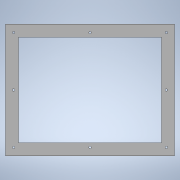
# Autodesk Inventor part: auth panel face plate seal
Saved by Autodesk Inventor 2022 (Build 260153000, 153)
## iProperties
Created: 2022-05-25
Part Number: auth panel face plate seal
Material: Generic
Document SubType Name: Modeling
Designer: alecw
Density: 1 g/cm^3
Appearance: Default
Author: alecw
Autodesk Inventor part; units mm, degrees
ref_plane "YZ Plane" through (0, 0, 0) normal (1, 0, 0) x (0, 1, 0)
ref_plane "XZ Plane" through (0, 0, 0) normal (0, 1, 0) x (-1, 0, 0)
ref_plane "Backplate Depth" through (0, 0, -3.2) normal (0, 0, 1) x (1, 0, 0)
sketch "Sketch2" plane through (0, 0, 0) normal (0, 0, 1) x (1, 0, 0)
  line L0 (0, 0) -> (49.8, 0)
  line L1 (49.8, 0) -> (49.8, 65)
  line L2 (49.8, 65) -> (0, 65)
  line L3 (0, 65) -> (0, 0)
  line L4 (0, 0) -> (-8.8, 0)
  line L5 (-8.8, 0) -> (-12, 0)
  line L6 (-12, 0) -> (-42, 0)
  line L7 (-42, 0) -> (-54.8, 0)
  line L8 (-54.8, 0) -> (-99.5, 0)
  line L9 (-99.5, 0) -> (-105.9, 0)
  line L10 (-105.9, 0) -> (-114.7, 0)
  line L11 (-114.7, 0) -> (-114.7, 40.1)
  line L12 (-114.7, 40.1) -> (0, 40.1)
  line L13 (-114.7, 0) -> (0, 0)
  line L14 (-105.9, 0) -> (-105.9, 40.1)
  line L15 (-8.8, 40.1) -> (-8.8, 0)
  line L16 (-48.4, 0) -> (-8.8, 0)
  line L17 (0, 65) -> (-114.7, 65)
  line L18 (-114.7, 65) -> (-114.7, 40.1)
  line L19 (49.8, 0) -> (54.6, 0)
  line L20 (0, 65) -> (0, 69.8)
  line L21 (0, 69.8) -> (54.6, 69.8)
  line L22 (54.6, 69.8) -> (54.6, 0)
  line L23 (-54.8, 0) -> (-48.4, 0)
  line L24 (-42, 0) -> (-48.4, 0)
  line L25 (-48.4, 0) -> (-48.4, 40.1)
  line L26 (-105.9, 40.1) -> (-105.9, 33.7)
  line L27 (-105.9, 40.1) -> (-93.1, 40.1)
  line L28 (-105.9, 0) -> (-48.4, 0)
  line L29 (-99.5, 0) -> (-88.19, 0)
  line L30 (-88.19, 0) -> (-79.22, 0)
  line L31 (-54.8, 0) -> (-54.8, 40.1)
  line L32 (-99.5, 0) -> (-99.5, 40.1)
  line L33 (-54.8, 40.1) -> (-56.9213, 37.9787)
  line L34 (-54.8, 40.1) -> (-51.8, 40.1) construction
  line L35 (-56.9213, 37.9787) -> (-54.8, 35.8574)
  line L36 (-56.9213, 37.9787) -> (-59.0426, 40.1)
  line L37 (-54.8, 0) -> (-57.6284, 2.8284)
  line L38 (-54.8, 0) -> (-50.8, 0) construction
  line L39 (-99.5, 40.1) -> (-95.9645, 36.5645)
  line L40 (-99.5, 40.1) -> (-94.5, 40.1) construction
  line L41 (-95.9645, 36.5645) -> (-92.4289, 40.1)
  line L42 (-95.9645, 36.5645) -> (-99.5, 33.0289)
  line L43 (-99.5, 0) -> (-95.9645, 3.5355)
  line L44 (-99.5, 0) -> (-94.5, 0) construction
  line L45 (-95.9645, 3.5355) -> (-92.4289, 0)
  line L46 (-95.9645, 3.5355) -> (-99.5, 7.0711)
  line L47 (-48.4, 0) -> (-48.4, -6.4)
  line L48 (-48.4, -6.4) -> (-105.9, -6.4)
  line L49 (-105.9, -6.4) -> (-105.9, 0)
  line L50 (-105.9, 40.1) -> (-105.9, 46.5)
  line L51 (-48.4, 40.1) -> (-48.4, 46.5)
  line L52 (-48.4, 46.5) -> (-105.9, 46.5)
  line L53 (-88.19, 0) -> (-86.59, 0)
  line L54 (-88.19, 0) -> (-89.79, 0)
  line L55 (-89.79, 0) -> (-86.59, 0)
  line L56 (-86.59, 0) -> (-86.59, 40.1)
  line L57 (-86.59, 40.1) -> (-89.79, 40.1)
  line L58 (-89.79, 40.1) -> (-89.79, 0)
  line L59 (-80.82, 40.1) -> (-80.82, 0)
  line L60 (-77.62, 0) -> (-77.62, 40.1)
  line L61 (-71.85, 40.1) -> (-71.85, 0)
  line L62 (-68.65, 0) -> (-68.65, 40.1)
  line L63 (-62.88, 40.1) -> (-62.88, 0)
  line L64 (-59.68, 0) -> (-59.68, 40.1)
  line L65 (0, 0) -> (0, -6.4)
  line L66 (0, -6.4) -> (0, -15.2)
  line L67 (-114.7, 0) -> (-114.7, -6.4)
  line L68 (-114.7, -6.4) -> (-114.7, -15.2)
  line L69 (-114.7, -15.2) -> (0, -15.2)
  line L70 (0, -15.2) -> (54.6, -15.2)
  line L71 (54.6, -15.2) -> (54.6, 0)
  line L72 (-28.6, 40.1) -> (-28.6, 0)
  circle A0 centre (-28.6, 20.05) radius 9.5
  circle A1 centre (-28.6, 20.05) radius 10.5
  line L73 (-28.6, 29.55) -> (-27.303, 29.4611)
  line L74 (-27.303, 29.4611) -> (-27.2345, 30.4608)
  line L75 (-28.6, 29.55) -> (-29.897, 29.4611)
  line L76 (-29.897, 29.4611) -> (-29.9655, 30.4608)
  line L77 (-105.9, 46.5) -> (-114.7, 46.5)
  line L78 (-105.9, -6.4) -> (-114.7, -6.4)
  line L79 (-48.4, -6.4) -> (0, -6.4)
  line L80 (-28.6, 20.05) -> (-35, 20.05)
  line L81 (-28.6, 20.05) -> (-22.2, 20.05)
  circle A2 centre (-28.6, 20.05) radius 14.7
  line L82 (-77.62, 40.1) -> (-71.85, 40.1)
  line L83 (-88.19, 40.1) -> (-92.19, 40.1)
  line L84 (-92.19, 40.1) -> (-93.79, 40.1)
  line L85 (-74.735, 0) -> (-74.735, 40.1)
  line L86 (-92.135, 38.25) -> (-57.335, 38.25)
  line L87 (-57.335, 38.25) -> (-57.335, 1.85)
  line L88 (-57.335, 1.85) -> (-92.135, 1.85)
  line L89 (-92.135, 1.85) -> (-92.135, 38.25)
  line L90 (-92.135, 38.25) -> (-57.335, 1.85) construction
  line L91 (-57.335, 38.25) -> (-92.135, 1.85) construction
  line L92 (-74.735, 38.25) -> (-74.735, 40.1)
  line L93 (-18.1, 20.05) -> (-17.1, 20.05)
  circle A3 centre (-28.6, 20.05) radius 11.5
  line L94 (-17.1, 20.05) -> (-13.9, 20.05)
  line L95 (-54.8, 40.1) -> (-48.4, 40.1)
  line L96 (-89.79, 38.25) -> (-86.59, 38.25)
  line L97 (-59.68, 38.25) -> (-62.88, 38.25)
  line L98 (-92.135, 20.05) -> (-57.335, 20.05)
  line L99 (-57.6284, 2.8284) -> (-54.8, 5.6569)
  line L100 (-57.6284, 2.8284) -> (-60.4569, 0)
  line L101 (-99.5, 20.05) -> (-105.9, 20.05)
  circle A4 centre (-102.7, 20.05) radius 0.9
  line L102 (-54.8, 20.05) -> (-48.4, 20.05)
  circle A5 centre (-51.6, 20.05) radius 0.9
  line L103 (0, -15.2) -> (0, -20)
  line L104 (0, -20) -> (-114.7, -20)
  line L105 (-114.7, -20) -> (-114.7, -15.2)
  line L106 (-88.19, 40.1) -> (-88.19, 43.3)
  circle A6 centre (-88.19, 43.3) radius 0.9
  circle A7 centre (-61.28, 43.3) radius 0.9
  line L107 (-102.7, 20.05) -> (-102.7, 0)
  circle A8 centre (-102.7, 10.025) radius 0.9
  circle A9 centre (-102.7, 30.075) radius 0.9
  circle A10 centre (-51.6, 30.075) radius 0.9
  circle A11 centre (-51.6, 10.025) radius 0.9
  line L108 (0, -20) -> (54.6, -20)
  line L109 (54.6, -20) -> (54.6, -15.2)
  line L110 (0, 65) -> (0, 73.8)
  line L111 (0, 73.8) -> (-114.7, 73.8)
  line L112 (-114.7, 73.8) -> (-114.7, 65)
  line L113 (-105.9, -20) -> (-105.9, 73.8)
  line L114 (-8.8, -20) -> (-8.8, 73.8)
  line L115 (-28.6, 40.1) -> (-48.4, 40.1)
  line L116 (-28.6, 40.1) -> (-8.8, 40.1)
  line L117 (-48.4, 46.5) -> (-28.6, 46.5)
  line L118 (-28.6, 46.5) -> (-8.8, 46.5)
  line L119 (-28.6, 46.5) -> (-28.6, 65)
  line L120 (-25.4, 52.55) -> (-31.8, 52.55)
  line L121 (-31.8, 52.55) -> (-31.8, 58.95)
  line L122 (-31.8, 58.95) -> (-25.4, 58.95)
  line L123 (-25.4, 58.95) -> (-25.4, 52.55)
  line L124 (-25.4, 52.55) -> (-31.8, 58.95) construction
  line L125 (-31.8, 52.55) -> (-25.4, 58.95) construction
  line L126 (-24.1, 51.25) -> (-33.1, 51.25)
  line L127 (-33.1, 51.25) -> (-33.1, 60.25)
  line L128 (-33.1, 60.25) -> (-24.1, 60.25)
  line L129 (-24.1, 60.25) -> (-24.1, 51.25)
  line L130 (-24.1, 51.25) -> (-33.1, 60.25) construction
  line L131 (-33.1, 51.25) -> (-24.1, 60.25) construction
  line L132 (-25.4, 52.55) -> (-25.4, 51.25)
  line L133 (-31.8, 52.55) -> (-31.8, 51.25)
  circle A12 centre (-88.19, 43.3) radius 2.4
  circle A13 centre (-61.28, 43.3) radius 2.4
  circle A14 centre (-51.6, 30.075) radius 2.4
  circle A15 centre (-51.6, 20.05) radius 2.4
  circle A16 centre (-102.7, 10.025) radius 2.4
  circle A17 centre (-102.7, 20.05) radius 2.4
  circle A18 centre (-102.7, 30.075) radius 2.4
  line L134 (-114.7, -20) -> (-114.7, -22.4)
  line L135 (-114.7, -22.4) -> (-117.1, -22.4)
  line L136 (-114.7, -15.2) -> (-114.7, -12.8)
  line L137 (-114.7, -12.8) -> (-112.3, -12.8)
  line L138 (0, 73.8) -> (-2.4, 73.8)
  line L139 (-2.4, 73.8) -> (-2.4, 71.4)
  line L140 (-112.3, -12.8) -> (-112.3, 71.4)
  line L141 (-112.3, 71.4) -> (-2.4, 71.4)
  line L142 (-2.4, 71.4) -> (-2.4, -12.8)
  line L143 (-2.4, -12.8) -> (-112.3, -12.8)
  line L144 (-2.4, -15.2) -> (-2.4, -12.8)
  line L145 (-28.6, -6.4) -> (-28.6, 0)
  circle A19 centre (-28.6, -3.2) radius 2.4
  circle A20 centre (-28.6, -3.2) radius 0.9
  line L146 (-28.6, 40.1) -> (-28.6, 46.5)
  circle A21 centre (-28.6, 43.3) radius 0.9
  circle A22 centre (-28.6, 43.3) radius 2.4
  line L147 (-105.9, 65) -> (-105.9, 71.4)
  circle A23 centre (-109.1, 68.2) radius 0.9
  circle A24 centre (-109.1, 68.2) radius 2
  line L148 (-8.8, 65) -> (-2.4, 65)
  line L149 (-8.8, -6.4) -> (-8.8, -12.8)
  line L150 (-105.9, 65) -> (-112.3, 65)
  line L151 (-105.9, 65) -> (-105.9, 71.4)
  line L152 (-105.9, 68.2) -> (-109.1, 68.2)
  line L153 (-109.1, 65) -> (-109.1, 68.2)
  line L154 (-105.9, -6.4) -> (-105.9, -12.8)
  circle A25 centre (-57.35, 68.2) radius 2
  circle A26 centre (-57.35, 68.2) radius 0.9
  circle A27 centre (-5.6, 68.2) radius 2
  circle A28 centre (-5.6, 68.2) radius 0.9
  circle A29 centre (-109.1, -9.6) radius 2
  circle A30 centre (-109.1, -9.6) radius 0.9
  circle A31 centre (-57.35, -9.6) radius 2
  circle A32 centre (-57.35, -9.6) radius 0.9
  circle A33 centre (-5.6, -9.6) radius 2
  circle A34 centre (-5.6, -9.6) radius 0.9
  line L155 (-105.9, -6.4) -> (-105.9, 65)
  line L156 (-105.9, 29.3) -> (-112.3, 29.3)
  circle A35 centre (-109.1, 29.3) radius 2
  circle A36 centre (-109.1, 29.3) radius 0.9
  circle A37 centre (-5.6, 29.3) radius 0.9
  circle A38 centre (-5.6, 29.3) radius 2
  line L157 (-105.9, 29.3) -> (-105.9, 65)
  line L158 (-8.8, 65) -> (-105.9, 65)
  line L159 (-57.35, 65) -> (-109.1, 65)
  circle A39 centre (-109.1, 68.2) radius 1.6
  circle A40 centre (-97.6, 68.2) radius 1.6
  circle A41 centre (-86.1, 68.2) radius 1.6
  circle A42 centre (-74.6, 68.2) radius 1.6
  circle A43 centre (-63.1, 68.2) radius 1.6
  circle A44 centre (-51.6, 68.2) radius 1.6
  circle A45 centre (-40.1, 68.2) radius 1.6
  circle A46 centre (-28.6, 68.2) radius 1.6
  circle A47 centre (-17.1, 68.2) radius 1.6
  circle A48 centre (-109.1, 57.0857) radius 1.6
  circle A49 centre (-109.1, 45.9714) radius 1.6
  circle A50 centre (-109.1, 34.8571) radius 1.6
  circle A51 centre (-109.1, 23.7429) radius 1.6
  circle A52 centre (-109.1, 12.6286) radius 1.6
  circle A53 centre (-109.1, 1.5143) radius 1.6
  line L160 (-57.35, 65) -> (-57.35, 71.4)
  circle A54 centre (-97.6, -9.6) radius 1.6
  circle A55 centre (-86.1, -9.6) radius 1.6
  circle A56 centre (-74.6, -9.6) radius 1.6
  circle A57 centre (-63.1, -9.6) radius 1.6
  circle A58 centre (-51.6, -9.6) radius 1.6
  circle A59 centre (-40.1, -9.6) radius 1.6
  circle A60 centre (-28.6, -9.6) radius 1.6
  circle A61 centre (-17.1, -9.6) radius 1.6
  circle A62 centre (-5.6, 57.0857) radius 1.6
  circle A63 centre (-5.6, 45.9714) radius 1.6
  circle A64 centre (-5.6, 34.8571) radius 1.6
  circle A65 centre (-5.6, 23.7429) radius 1.6
  circle A66 centre (-5.6, 12.6286) radius 1.6
  circle A67 centre (-5.6, 1.5143) radius 1.6
  line L161 (-48.4, 46.5) -> (-48.4, 65)
  line L162 (-92.135, 38.25) -> (-92.985, 38.25)
  line L163 (-92.985, 38.25) -> (-92.985, 39.1)
  line L164 (-56.485, 1) -> (-92.985, 1)
  line L165 (-92.985, 1) -> (-92.985, 39.1)
  line L166 (-92.985, 39.1) -> (-56.485, 39.1)
  line L167 (-56.485, 39.1) -> (-56.485, 1)
  line L168 (-56.485, 1) -> (-92.985, 39.1) construction
  line L169 (-92.985, 1) -> (-56.485, 39.1) construction
  line L170 (-92.985, 39.1) -> (-92.985, 40.1)
  line L171 (-92.985, 40.1) -> (-93.985, 40.1)
  line L172 (-55.485, 0) -> (-93.985, 0)
  line L173 (-93.985, 0) -> (-93.985, 40.1)
  line L174 (-93.985, 40.1) -> (-55.485, 40.1)
  line L175 (-55.485, 40.1) -> (-55.485, 0)
  line L176 (-55.485, 0) -> (-93.985, 40.1) construction
  line L177 (-93.985, 0) -> (-55.485, 40.1) construction
  line L178 (54.6, -20) -> (59.6, -20)
  line L179 (59.6, -20) -> (59.6, 69.8)
  line L180 (59.6, 69.8) -> (54.6, 69.8)
  line L181 (59.6, -20) -> (61.6, -20)
  line L182 (61.6, -20) -> (61.6, 69.8)
  line L183 (61.6, 69.8) -> (59.6, 69.8)
  line L184 (59.6, 65) -> (61.6, 65)
  line L185 (59.6, -20) -> (59.6, -16.8)
  line L186 (59.6, -16.8) -> (61.6, -16.8)
  line L187 (-8.8, -20) -> (-105.9, -20)
  line L188 (-105.9, -20) -> (-101.9, -20)
  line L189 (-57.35, -20) -> (-57.35, -15.2)
  line L190 (-101.9, -20) -> (-101.4, -20)
  line L191 (-101.4, -20) -> (-93.4, -20)
  line L192 (-93.4, -20) -> (-93.4, -15.2)
  line L193 (-101.9, -20) -> (-101.9, -15.2)
  line L194 (-101.4, -20) -> (-101.4, -15.2)
  line L195 (-93.4, -20) -> (-92.9, -20)
  line L196 (-92.9, -20) -> (-84.9, -20)
  line L197 (-84.9, -20) -> (-84.9, -15.2)
  line L198 (-8.8, -20) -> (-12.8, -20)
  line L199 (-12.8, -20) -> (-13.3, -20)
  line L200 (-13.3, -20) -> (-21.3, -20)
  line L201 (-21.3, -20) -> (-21.3, -15.2)
  line L202 (-12.8, -20) -> (-12.8, -15.2)
  line L203 (-13.3, -20) -> (-13.3, -15.2)
  line L204 (-21.3, -20) -> (-21.8, -20)
  line L205 (-21.8, -20) -> (-29.8, -20)
  line L206 (-29.8, -20) -> (-29.8, -15.2)
  line L207 (-57.35, 73.8) -> (-57.35, 75.8)
  line L208 (-57.35, 75.8) -> (-77.35, 75.8)
  line L209 (-77.35, 75.8) -> (-79.35, 73.8)
  line L210 (-77.35, 75.8) -> (-74.5216, 75.8) construction
  line L211 (-57.35, 75.8) -> (-37.35, 75.8)
  line L212 (-37.35, 75.8) -> (-35.35, 73.8)
  line L213 (0, 73.8) -> (61.6, 73.8)
  line L214 (61.6, 73.8) -> (61.6, 69.8)
  line L215 (0, 73.8) -> (0.5, 73.8)
  line L216 (0.5, 73.8) -> (0.5, -20)
  line L217 (59.6, 69.8) -> (59.6, 73.8)
  line L218 (54.6, -15.2) -> (61.6, -15.2)
  line L219 (-92.9, -20) -> (-92.9, -15.2)
  line L220 (-21.8, -20) -> (-21.8, -15.2)
  line L221 (0.5, -15.2) -> (0.5, -10.4)
  line L222 (0.5, -10.4) -> (54.6, -10.4)
  line L223 (0.5, -15.2) -> (0.5, -10.4)
  line L224 (0.5, -10.4) -> (54.6, -10.4)
  line L225 (49.8, 0) -> (49.8, -15.2)
  line L226 (49.8, 69.8) -> (49.8, 65)
  line L227 (54.6, 65) -> (49.8, 65)
  line L228 (0.5, -15.2) -> (5.3, -15.2)
  line L229 (5.3, -15.2) -> (5.3, 65)
  line L230 (54.6, 69.8) -> (54.6, 73.8)
  line L231 (49.8, 69.8) -> (49.8, 73.8)
  line L232 (49.8, -15.2) -> (49.8, -20)
  line L233 (5.3, -15.2) -> (5.3, -20)
  line L234 (5.3, 65) -> (5.3, 73.8)
  line L235 (54.6, -10.4) -> (61.6, -10.4)
  line L236 (61.6, 65) -> (54.6, 65)
  line L237 (-35, 20.05) -> (-35, 13.0293)
  line L238 (-35, 20.05) -> (-35, 27.0707)
  line L239 (-22.2, 20.05) -> (-22.2, 27.0707)
  line L240 (-22.2, 20.05) -> (-22.2, 13.0293)
  line L241 (0, -6.4) -> (61.6, -6.4)
  line L242 (0, 0) -> (61.6, 0)
  line L243 (-35, 27.0707) -> (-35, 33.2837)
  line L244 (-22.2, 27.0707) -> (-22.2, 33.2837)
  line L245 (-27.303, 10.6389) -> (-27.2345, 9.6392)
  line L246 (-29.897, 10.6389) -> (-29.9655, 9.6392)
  line L247 (-35, 20.05) -> (-35, 6.8163)
  line L248 (-22.2, 20.05) -> (-22.2, 6.8163)
  line L249 (-99.5, 33.0289) -> (-101.5, 33.0289)
  line L250 (-92.4289, 40.1) -> (-92.4289, 42.1)
  line L251 (-92.4289, 42.1) -> (-101.5, 42.1)
  line L252 (-101.5, 42.1) -> (-101.5, 33.0289)
  line L253 (-99.5, 7.0711) -> (-101.5, 7.0711)
  line L254 (-92.4289, 0) -> (-92.4289, -2)
  line L255 (-92.4289, -2) -> (-101.5, -2)
  line L256 (-101.5, -2) -> (-101.5, 7.0711)
  line L257 (-54.8, 5.6569) -> (-52.8, 5.6569)
  line L258 (-60.4569, 0) -> (-60.4569, -2)
  line L259 (-60.4569, -2) -> (-52.8, -2)
  line L260 (-52.8, -2) -> (-52.8, 5.6569)
  line L261 (-59.0426, 40.1) -> (-59.0426, 42.1)
  line L262 (-54.8, 35.8574) -> (-52.8, 35.8574)
  line L263 (-52.8, 35.8574) -> (-52.8, 42.1)
  line L264 (-52.8, 42.1) -> (-59.0426, 42.1)
  line L265 (-28.6, 52.55) -> (-30.1, 52.55)
  line L266 (-30.1, 52.55) -> (-30.1, 51.25)
  line L267 (-28.6, 52.55) -> (-27.1, 52.55)
  line L268 (-27.1, 52.55) -> (-27.1, 51.25)
  line L269 (-2.4, 29.3) -> (-2.4, 32.5)
  line L270 (-2.4, 32.5) -> (-8.8, 32.5)
  line L271 (-2.4, 29.3) -> (-2.4, 26.1)
  line L272 (-2.4, 26.1) -> (-8.8, 26.1)
  line L273 (-27.1, 58.95) -> (-27.1, 60.25)
  line L274 (-30.1, 58.95) -> (-30.1, 60.25)
  line L275 (-31.8, 58.95) -> (-31.8, 62.15)
  line L276 (-31.8, 62.15) -> (-35, 62.15)
  line L277 (-22.2, 49.35) -> (-35, 49.35)
  line L278 (-35, 49.35) -> (-35, 62.15)
  line L279 (-35, 62.15) -> (-22.2, 62.15)
  line L280 (-22.2, 62.15) -> (-22.2, 49.35)
  line L281 (-22.2, 49.35) -> (-35, 62.15) construction
  line L282 (-35, 49.35) -> (-22.2, 62.15) construction
  line L283 (-31.8, 58.95) -> (-32.1, 58.95)
  line L284 (-32.1, 58.95) -> (-32.1, 59.25)
  line L285 (-25.1, 52.25) -> (-32.1, 52.25)
  line L286 (-32.1, 52.25) -> (-32.1, 59.25)
  line L287 (-32.1, 59.25) -> (-25.1, 59.25)
  line L288 (-25.1, 59.25) -> (-25.1, 52.25)
  line L289 (-25.1, 52.25) -> (-32.1, 59.25) construction
  line L290 (-32.1, 52.25) -> (-25.1, 59.25) construction
  line L291 (-28.6, 55.75) -> (-28.6, 52.55)
  line L292 (-44.6, 52.55) -> (-38.2, 52.55)
  line L293 (-38.2, 52.55) -> (-38.2, 58.95)
  line L294 (-38.2, 58.95) -> (-44.6, 58.95)
  line L295 (-44.6, 58.95) -> (-44.6, 52.55)
  line L296 (-44.6, 52.55) -> (-38.2, 58.95) construction
  line L297 (-38.2, 52.55) -> (-44.6, 58.95) construction
  line L298 (-45.9, 51.25) -> (-36.9, 51.25)
  line L299 (-36.9, 51.25) -> (-36.9, 60.25)
  line L300 (-36.9, 60.25) -> (-45.9, 60.25)
  line L301 (-45.9, 60.25) -> (-45.9, 51.25)
  line L302 (-45.9, 51.25) -> (-36.9, 60.25) construction
  line L303 (-36.9, 51.25) -> (-45.9, 60.25) construction
  line L304 (-44.6, 52.55) -> (-44.6, 51.25)
  line L305 (-38.2, 52.55) -> (-38.2, 51.25)
  line L306 (-41.4, 52.55) -> (-39.9, 52.55)
  line L307 (-39.9, 52.55) -> (-39.9, 51.25)
  line L308 (-41.4, 52.55) -> (-42.9, 52.55)
  line L309 (-42.9, 52.55) -> (-42.9, 51.25)
  line L310 (-42.9, 58.95) -> (-42.9, 60.25)
  line L311 (-39.9, 58.95) -> (-39.9, 60.25)
  line L312 (-38.2, 58.95) -> (-38.2, 62.15)
  line L313 (-38.2, 62.15) -> (-35, 62.15)
  line L314 (-47.8, 49.35) -> (-35, 49.35)
  line L315 (-35, 62.15) -> (-47.8, 62.15)
  line L316 (-47.8, 62.15) -> (-47.8, 49.35)
  line L317 (-47.8, 49.35) -> (-35, 62.15) construction
  line L318 (-35, 49.35) -> (-47.8, 62.15) construction
  line L319 (-38.2, 58.95) -> (-37.9, 58.95)
  line L320 (-37.9, 58.95) -> (-37.9, 59.25)
  line L321 (-44.9, 52.25) -> (-37.9, 52.25)
  line L322 (-37.9, 52.25) -> (-37.9, 59.25)
  line L323 (-37.9, 59.25) -> (-44.9, 59.25)
  line L324 (-44.9, 59.25) -> (-44.9, 52.25)
  line L325 (-44.9, 52.25) -> (-37.9, 59.25) construction
  line L326 (-37.9, 52.25) -> (-44.9, 59.25) construction
  line L327 (-41.4, 55.75) -> (-41.4, 52.55)
  line L328 (-15.8, 46.5) -> (-15.8, 65)
  line L329 (-19, 52.55) -> (-12.6, 52.55)
  line L330 (-12.6, 52.55) -> (-12.6, 58.95)
  line L331 (-12.6, 58.95) -> (-19, 58.95)
  line L332 (-19, 58.95) -> (-19, 52.55)
  line L333 (-19, 52.55) -> (-12.6, 58.95) construction
  line L334 (-12.6, 52.55) -> (-19, 58.95) construction
  line L335 (-20.3, 51.25) -> (-11.3, 51.25)
  line L336 (-11.3, 51.25) -> (-11.3, 60.25)
  line L337 (-11.3, 60.25) -> (-20.3, 60.25)
  line L338 (-20.3, 60.25) -> (-20.3, 51.25)
  line L339 (-20.3, 51.25) -> (-11.3, 60.25) construction
  line L340 (-11.3, 51.25) -> (-20.3, 60.25) construction
  line L341 (-19, 52.55) -> (-19, 51.25)
  line L342 (-12.6, 52.55) -> (-12.6, 51.25)
  line L343 (-15.8, 52.55) -> (-14.3, 52.55)
  line L344 (-14.3, 52.55) -> (-14.3, 51.25)
  line L345 (-15.8, 52.55) -> (-17.3, 52.55)
  line L346 (-17.3, 52.55) -> (-17.3, 51.25)
  line L347 (-17.3, 58.95) -> (-17.3, 60.25)
  line L348 (-14.3, 58.95) -> (-14.3, 60.25)
  line L349 (-12.6, 58.95) -> (-12.6, 62.15)
  line L350 (-12.6, 62.15) -> (-9.4, 62.15)
  line L351 (-22.2, 49.35) -> (-9.4, 49.35)
  line L352 (-9.4, 49.35) -> (-9.4, 62.15)
  line L353 (-9.4, 62.15) -> (-22.2, 62.15)
  line L354 (-22.2, 49.35) -> (-9.4, 62.15) construction
  line L355 (-9.4, 49.35) -> (-22.2, 62.15) construction
  line L356 (-12.6, 58.95) -> (-12.3, 58.95)
  line L357 (-12.3, 58.95) -> (-12.3, 59.25)
  line L358 (-19.3, 52.25) -> (-12.3, 52.25)
  line L359 (-12.3, 52.25) -> (-12.3, 59.25)
  line L360 (-12.3, 59.25) -> (-19.3, 59.25)
  line L361 (-19.3, 59.25) -> (-19.3, 52.25)
  line L362 (-19.3, 52.25) -> (-12.3, 59.25) construction
  line L363 (-12.3, 52.25) -> (-19.3, 59.25) construction
  line L364 (-15.8, 55.75) -> (-15.8, 52.55)
  line L365 (-77.15, 46.5) -> (-77.15, 65)
  line L366 (5.3, -15.2) -> (5.3, -10.4)
  line L367 (0.5, -10.4) -> (5.3, -10.4)
  line L368 (5.3, -12.8) -> (2.9, -12.8)
  line L369 (2.9, -12.8) -> (2.9, -10.4)
  circle A68 centre (2.9, -12.8) radius 1
  circle A69 centre (2.9, -12.8) radius 0.9
  line L370 (54.6, -10.4) -> (49.8, -10.4)
  line L371 (52.2, -10.4) -> (2.9, -10.4)
  line L372 (5.3, 66.25) -> (5.3, -12.8)
  circle A70 centre (2.9, -12.8) radius 1.6
  line L373 (5.3, 69.8) -> (5.3, 65)
  line L374 (5.3, 67.4) -> (5.3, -12.8)
  line L375 (2.9, -10.4) -> (52.2, -10.4)
  point P0 (-74.735, 20.05)
  point P1 (-74.735, 20.05)
  point P2 (-112.3, 0)
  point P3 (-8.8, 71.4)
  point P4 (0.5, 0)
  point P5 (0, 69.8)
  point P6 (59.6, -15.2)
  point P7 (-8.8, -15.2)
  point P8 (-105.9, -15.2)
  point P9 (5.3, 0)
  point P10 (54.6, 0)
  point P11 (59.6, 0)
  point P12 (59.6, 65)
  point P13 (-60.4569, 0)
  point P14 (-60.4569, 0)
  point P15 (-92.4289, 0)
  point P16 (-68.65, 38.25)
  point P17 (-71.85, 38.25)
  point P18 (-71.85, 1.85)
  point P19 (-68.65, 1.85)
  point P20 (-62.88, 1.85)
  point P21 (-59.68, 1.85)
  point P22 (-80.82, 1.85)
  point P23 (-77.62, 1.85)
  point P24 (-77.62, 38.25)
  point P25 (-80.82, 38.25)
  point P26 (-86.59, 38.25)
  point P27 (-89.79, 1.85)
  point P28 (-86.59, 1.85)
  point P29 (-92.4289, 0)
  point P30 (-60.4569, 0)
  point P31 (49.8, -6.4)
  point P32 (5.3, -6.4)
  dimension "d1" = 49.8
  dimension "d2" = 65
  dimension "d3" = 8.8
  dimension "d4" = 3.2
  dimension "d5" = 30
  dimension "d6" = 12.8
  dimension "d7" = 44.7
  dimension "d11" = 40.1
  dimension "d15" = 4.8
  dimension "d16" = 4.8
  dimension "d21" = 11.31
  dimension "d22" = 8.97
  dimension "d23" = 3
  dimension "d24" = 135
  dimension "d25" = 4
  dimension "d26" = 135
  dimension "d27" = 5
  dimension "d28" = 45
  dimension "d29" = 5
  dimension "d30" = 45
  dimension "d33" = 6.4
  dimension "d34" = 1.6
  dimension "d35" = 1.6
  dimension "d38" = 8.97
  dimension "d43" = 3.2
  dimension "d45" = 19
  dimension "d46" = 21
  dimension "d47" = 1.3
  dimension "d48" = 6.4
  dimension "d49" = 6.4
  dimension "d53" = 4
  dimension "d54" = 1.6
  dimension "d55" = 34.8
  dimension "d56" = 36.4
  dimension "d59" = 1
  dimension "d61" = 3.2
  dimension "d70" = 1.8
  dimension "d71" = 1.8
  dimension "d72" = 4.8
  dimension "d74" = 3.2
  dimension "d75" = 1.8
  dimension "d76" = 1.8
  dimension "d79" = 51.1
  dimension "d86" = 6.4
  dimension "d88" = 9
  dimension "d89" = 4.8
  dimension "d98" = 2.4
  dimension "d99" = 2.4
  dimension "d100" = 2.4
  dimension "d101" = 2.4
  dimension "d102" = 2.4
  dimension "d103" = 2.4
  dimension "d104" = 2.4
  dimension "d105" = 1.8
  dimension "d106" = 4
  dimension "d109" = 51.75
  dimension "d116" = 77.8
  dimension "d123" = 38.9
  dimension "d128" = 3.2
  dimension "d131" = 11.5
  dimension "d138" = 11.1143
  dimension "d143" = 0.85
  dimension "d144" = 0.85
  dimension "d145" = 1
  constraints: 748 end point, 146 point on line, 94 symmetric about line, 71 centre point, 70 perpendicular, 65 midpoint, 55 horizontal, 45 vertical, 37 parallel, 26 coincident, 23 collinear, 15 point on circle, 14 horizontal alignment, 12 equal radius, 5 equal length, 96 other
  measures "d1" distance of L2.end L1.end
  measures "d2" distance of L1.end L0.end
  measures "d3" distance of L0.start L4.end
  measures "d4" distance of L4.end L5.end
  measures "d5" distance of L5.end L6.end
  measures "d6" distance of L6.end L7.end
  measures "d7" distance of L7.end L8.end
  measures "d11" distance of L10.end L11.end
  measures "d15" distance of L0.end L19.end
  measures "d16" distance of L2.end L20.end
  measures "d21" distance of L8.end L29.end
  measures "d22" distance of L29.end L30.end
  measures "d23" distance of L31.end L33.end
  measures "d24" angle of L33 L34
  measures "d25" distance of L7.end L37.end
  measures "d26" angle of L38 L37
  measures "d27" distance of L32.end L39.end
  measures "d28" angle of L39 L40
  measures "d29" distance of L8.end L43.end
  measures "d30" angle of L44 L43
  measures "d33" distance of L25.end L51.end
  measures "d34" distance of L29.end L53.end
  measures "d35" distance of L29.end L54.end
  measures "d38" distance of L57.end L59.start
  measures "d43" distance between parallel lines of L56 L58
  measures "d45" diameter of A0
  measures "d46" diameter of A1
  measures "d47" distance of L73.start L73.end
  measures "d48" distance of L80.start L80.end
  measures "d49" distance of L80.start L81.end
  measures "d53" distance of L83.start L83.end
  measures "d54" distance of L83.end L84.end
  measures "d55" distance of L87.end L88.end
  measures "d56" distance of L86.end L87.end
  measures "d59" distance of L93.start L93.end
  measures "d61" distance of L94.start L94.end
  measures "d70" diameter of A4
  measures "d71" diameter of A5
  measures "d72" distance of L66.end L103.end
  measures "d74" distance of L83.start L106.end
  measures "d75" diameter of A6
  measures "d76" diameter of A8
  measures "d79" distance of A9.centre A10.centre
  measures "d86" distance of L121.end L122.end
  measures "d88" distance of L126.end L127.end
  measures "d89" diameter of A12
  measures "d98" distance of L104.end L134.end
  measures "d99" distance of L134.end L135.end
  measures "d100" distance of L68.end L136.end
  measures "d101" distance of L136.end L137.end
  measures "d102" distance of L110.end L138.end
  measures "d103" distance of L138.end L139.end
  measures "d104" distance of L144.start L142.end
  measures "d105" diameter of A23
  measures "d106" diameter of A24
  measures "d109" distance of L152.end A25.centre
  measures "d116" distance of L152.end A29.centre
  measures "d123" distance of L152.end A35.centre
  measures "d128" diameter of A39
  measures "d131" distance of A39.centre A40.centre
  measures "d138" distance of A39.centre A48.centre
  measures "d143" distance of L86.start L162.end
  measures "d144" distance of L162.end L163.end
  measures "d145" distance of L163.end L170.end
ref_plane "Face Plate Start" through (0, 0, 5) normal (0, 0, 1) x (1, 0, 0)
ref_plane "TPU Seal Start" through (0, 0, 4) normal (0, 0, 1) x (1, 0, 0)
ref_plane "Face Plate End" through (0, 0, 8.2) normal (0, 0, 1) x (1, 0, 0)
ref_plane "Cover Clearance" through (0, 0, 11.2) normal (0, 0, 1) x (1, 0, 0)
ref_plane "Cover End" through (0, 0, 13.6) normal (0, 0, 1) x (1, 0, 0)
ref_plane "RFID Cover Start" through (0, 0, 12) normal (0, 0, 1) x (1, 0, 0)
extrude "Extrusion17" add sketch "Sketch2" along normal blind 0.6 contours L4 L142 L12 L3 | L65 L79 L142 L4 | L12 L142 L17 L3 | L142 L79 L114 L4 A67 | L4 A67 L15 L272 L142 | L66 L69 L144 L142 L79 | L17 L142 L139 L111 L110 L20 | L142 L270 L15 L12 | L12 L114 L17 L142 | A67 L4 | L4 A67 | L272 L15 L270 L142 | L142 L143 L114 L79 | L17 L114 L141 L142 | L114 L143 L113 L48 L79 | L144 L69 L114 L143 | L17 L160 A25 L141 L114 | L141 L114 L111 L139 | L114 L69 L113 L143 | L141 L113 L111 L114 | L143 L140 L78 L113 | L113 L69 L68 L137 L143 | L160 A25 L17 L113 L141 | L78 L140 L10 A53 L49 | L137 L68 L78 L140 | L141 L140 L17 L112 L111 L113 | L113 L152 A24 L153 L17 L140 L141 | L160 A26 A25 | A25 L160 A26 | L10 A53 L140 L156 A35 L14 | L78 L67 L10 L140 | L113 L17 L153 A24 L152 | L50 L12 L140 L77 A49 | L77 A49 L140 L17 L113 | A53 L10 | L10 A53 | L10 L11 L12 L140 | L152 A39 L153 A24 | A24 L153 A39 L152 | L140 L77 L18 L17 | L14 L156 A35 L140 L12 | A49 L77 | L77 A49 | A39 L153 A23 L152 | L152 A23 L153 A39 | L140 L12 L18 L77 | A35 L156 A36 | L156 A36 A35 | A27 | A29 | A31 | A33 | A38 | A40 | A41 | A42 | A43 | A44 | A45 | A46 | A47 | A48 | A50 | A51 | A52 | A54 | A55 | A56 | A57 | A58 | A59 | A60 | A61 | A62 | A63 | A64 | A65 | A66
body "Solid3"
